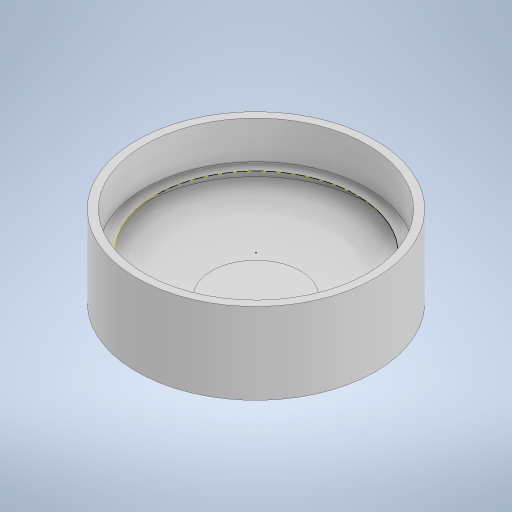
# Autodesk Inventor part: befor
Saved by Autodesk Inventor 2023 (Build 270158000, 158)
## iProperties
Created: 2023-09-22
Part Number: befor
Material: Generic
Document SubType Name: Modeling
Designer: 1908174
Density: 1 g/cm^3
Appearance: Default
Author: 1908174
Autodesk Inventor part; units mm, degrees
ref_plane "YZ Plane" through (0, 0, 0) normal (1, 0, 0) x (0, 1, 0)
ref_plane "XZ Plane" through (0, 0, 0) normal (0, 1, 0) x (-1, 0, 0)
ref_plane "XY Plane" through (0, 0, 0) normal (0, 0, 1) x (1, 0, 0)
sketch "Sketch1" plane through (0, 0, 0) normal (0, 1, 0) x (-1, 0, 0)
  circle A0 centre (0, 0) radius 16.002
  dimension "d0" = 32.004
  constraints: 1 centre point, 1 coincident
  measures "d0" diameter of A0
extrude "Extrusion1" add sketch "Sketch1" along normal blind 6.3246
sketch "Sketch2" plane through (0, 6.3246, 0) normal (0, 1, 0) x (1, 0, 0)
  circle A0 centre (0, 0) radius 13.335
  dimension "d3" = 26.67
  constraints: 1 centre point, 1 coincident
  measures "d3" diameter of A0
extrude "Extrusion2" add sketch "Sketch2" along normal blind 1.1176
fillet "Fillet1" radius 2.54 1 edges at (16.002, 6.3246, 0)
fillet "Fillet2" radius 15.24 1 edges at (16.002, 0, 0)
fillet "Fillet3" radius 0.254 1 edges at (-13.335, 7.4422, 0)
shell "Shell1" thickness 0.635 removed faces 3 at (13.1616, 7.2072, 2.139) at (13.2918, 6.9003, 1.073) at (2.477, 7.4422, -4.5655)
sketch "Sketch3" plane through (0, 0.635, 0) normal (0, 1, 0) x (1, 0, 0)
  circle A0 centre (0, 0) radius 5.9506
  constraints: 1 centre point, 1 coincident
extrude "Extrusion3" cut sketch "Sketch3" against normal blind 25.4
extrude "Extrusion4" add sketch "Sketch3" against normal blind 0.762
sketch "Sketch5" plane through (0, -0.127, 0) normal (0, -1, 0) x (1, 0, 0)
  circle A0 centre (0, 0) radius 16.002
  constraints: 1 centre point, 1 coincident
extrude "Extrusion6" add sketch "Sketch5" against normal up to next
sketch "Sketch7" plane through (0, 5.6896, 0) normal (0, -1, 0) x (1, 0, 0)
  circle A0 centre (0, 0) radius 15.3471
  circle A1 centre (0, 0) radius 16.002
  constraints: 2 centre point, 1 coincident
extrude "Extrusion7" add sketch "Sketch7" against normal blind 5.08 contours A0 | A1
sketch "Sketch8" plane through (0, 10.7696, 0) normal (0, 1, 0) x (1, 0, 0)
  circle A0 centre (0, 0) radius 14.9515
  constraints: 1 centre point, 1 coincident
extrude "Extrusion8" cut sketch "Sketch8" against normal blind 5.08
sketch "Sketch9" plane through (0, 5.6896, 0) normal (0, -1, 0) x (1, 0, 0)
  circle A0 centre (0, 0) radius 16.002
  circle A1 centre (0, 0) radius 15.1054
  constraints: 2 centre point, 2 coincident
extrude "Extrusion9" add sketch "Sketch9" along normal blind 4.7625
sketch "Sketch11" plane through (0, 5.6896, 0) normal (0, 1, 0) x (1, 0, 0)
  circle A0 centre (0, 0) radius 13.462 projected
  arc A1 (0, 13.462) -> (-13.462, 0) centre (0, 0) ccw
  arc A2 (13.462, 0) -> (0, 13.462) centre (0, 0) ccw
  arc A3 (-0.0694, -13.4618) -> (13.462, 0) centre (0, 0) ccw
  constraints: 10 point on circle, 4 concentric, 3 centre point
body "Solid1"
